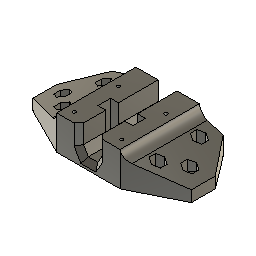
2Box Snare Int Bracket v1 (Autodesk Fusion 360 design; units mm, degrees)
Autodesk Fusion 360 part; units mm, degrees
sketch "Sketch1" plane through (0, 0, 0) normal (0, 0, 1) x (1, 0, 0)
  line L0 (0, 0) -> (40, 0)
  line L1 (40, 0) -> (40, 40)
  line L2 (40, 40) -> (0, 40)
  line L3 (0, 40) -> (0, 0)
  dimension "d1" = 40
  dimension "d2" = 40
  constraint horizontal L0
  constraint vertical L1
  constraint horizontal L2
  constraint vertical L3
  constraint coincident L0.start L3.end
  measures "d1" distance of L0.start L0.end
  measures "d2" distance of L0.start L2.end
extrude "Extrude1" add sketch "Sketch1" along normal blind 21.5
sketch "Sketch2" plane through (0, 0, 21.5) normal (0, 0, 1) x (-1, 0, 0)
  line L0 (0, -40) -> (0, 0)
  line L1 (0, 0) -> (-40, 0)
  line L2 (-40, 0) -> (-40, -40)
  line L3 (-40, -40) -> (0, -40)
  line L4 (-20, -55) -> (-20, 20) construction
  line L5 (-14.5, -40) -> (-25.5, -40)
  line L6 (-25.5, -40) -> (-25.5, 0)
  line L7 (-25.5, 0) -> (-14.5, 0)
  line L8 (-14.5, 0) -> (-14.5, -40)
  dimension "d5" = 20
  dimension "d6" = 11
  dimension "d7" = 5.5
  constraint perpendicular L3 L4
  constraint horizontal L5
  constraint vertical L6
  constraint horizontal L7
  constraint vertical L8
  constraint coincident L3 L5.start
  measures "d5" distance of L2 L4
  measures "d6" distance of L5.start L5.end
  measures "d7" distance of L4 L8
extrude "Extrude2" cut sketch "Sketch2" against normal blind 17 contours L1 L3 L5 L6 L7 L8
extrude "Extrude3" add 1 faces at (35.1667, 40, 8.6667) along direction (0, 1, 0) blind 10
sketch "Sketch3" plane through (0, 0, 0) normal (0, -1, 0) x (1, 0, 0)
  line L0 (25.5, 21.5) -> (25.5, 4.5)
  line L1 (25.5, 4.5) -> (14.5, 4.5)
  line L2 (14.5, 4.5) -> (14.5, 21.5)
  line L3 (14.5, 21.5) -> (0, 21.5)
  line L4 (0, 21.5) -> (0, 0)
  line L5 (0, 0) -> (40, 0)
  line L6 (40, 0) -> (40, 21.5)
  line L7 (40, 21.5) -> (25.5, 21.5)
  line L8 (13.9749, 9.6962) -> (16.9749, 4.5)
  line L9 (16.9749, 4.5) -> (22.9749, 4.5)
  line L10 (22.9749, 4.5) -> (25.9749, 9.6962)
  line L11 (14.5, 4.5) -> (30, 4.5) construction
  line L12 (25.9749, 9.6962) -> (25.9749, 21.5)
  line L13 (13.9749, 9.6962) -> (13.9749, 21.5)
  line L14 (13.9749, 21.5) -> (25.9749, 21.5)
  point P0 (19.9749, 9.6962)
  dimension "d13" = 12
  constraint coincident L1.end L2.start
  constraint perpendicular L2 L11
  constraint collinear L9 L11
  constraint coincident L7 L12.end
  constraint perpendicular L7 L12
  constraint coincident L3 L13.end
  constraint perpendicular L3 L13
  measures "d13" distance of L10.end L8.start
extrude "Extrude4" add 1 faces at (18.1667, 33.3333, 4.5) along direction (0, 0, 1) blind 17
extrude "Extrude5" cut sketch "Sketch3" against normal blind 61 contours L0 L7 L10 L12 L14 | L0 L1 L2 L8 L9 L10 L14 | L2 L3 L8 L13 L14
sketch "Sketch5" plane through (0, 0, 0) normal (0, 0, -1) x (1, 0, 0)
  line L0 (0, 0) -> (0, -50)
  line L1 (0, -50) -> (40, -50)
  line L2 (40, -50) -> (40, 0)
  line L3 (40, 0) -> (0, 0)
  circle A0 centre (20, -21) radius 4.5
  dimension "d19" = 9
  dimension "d20" = 21
  dimension "d21" = 20
  measures "d19" diameter of A0
  measures "d20" distance of L3 A0.centre
  measures "d21" distance of L2 A0.centre
extrude "Extrude6" cut sketch "Sketch5" against normal blind 51 contours A0
sketch "Sketch6" plane through (0, 0, 21.5) normal (0, 0, 1) x (-1, 0, 0)
  line L0 (-13.9749, 0) -> (-13.9749, -50)
  line L1 (-13.9749, -50) -> (0, -50)
  line L2 (0, -50) -> (0, 0)
  line L3 (0, 0) -> (-13.9749, 0)
  line L4 (-9, -25) -> (-31, -25)
  line L5 (-31, -25) -> (-31, -17)
  line L6 (-31, -17) -> (-9, -17)
  line L7 (-9, -17) -> (-9, -25)
  line L8 (-20, -32) -> (-20, 7) construction
  line L9 (4, -21) -> (-49, -21) construction
  dimension "d24" = 22
  dimension "d25" = 8
  dimension "d26" = 11
  dimension "d27" = 21
  dimension "d28" = 20
  dimension "d29" = 4
  constraint horizontal L4
  constraint vertical L5
  constraint horizontal L6
  constraint vertical L7
  constraint perpendicular L4 L8
  constraint perpendicular L5 L9
  measures "d24" distance of L4.start L4.end
  measures "d25" distance of L4.start L6.end
  measures "d26" distance of L7 L8
  measures "d27" distance of L3 L9
  measures "d28" distance of L2 L8
  measures "d29" distance of L4 L9
extrude "Extrude7" cut sketch "Sketch6" against normal blind 19 contours L0 L4 L6 L7 | L0 L4 L5 L6
sketch "Sketch7" plane through (0, 0, 0) normal (-1, 0, 0) x (0, -1, 0)
  line L0 (-50, 0) -> (0, 0)
  line L1 (0, 0) -> (0, 21.5)
  line L2 (0, 21.5) -> (-50, 21.5)
  line L3 (-50, 21.5) -> (-50, 0)
  line L4 (-50, 0) -> (0, 0)
  line L5 (0, 0) -> (0, 15)
  line L6 (0, 15) -> (-50, 15)
  line L7 (-50, 15) -> (-50, 0)
  constraint horizontal L4
  constraint vertical L5
  constraint horizontal L6
  constraint vertical L7
  constraint coincident L1 L5.end
  constraint coincident L0.start L3.end
extrude "Extrude8" add sketch "Sketch7" along normal blind 30 contours L0 L1 L3 L4 L5 L6 L7
sketch "Sketch8" plane through (40, 0, 0) normal (1, 0, 0) x (0, 1, 0)
  line L0 (0, 0) -> (50, 0)
  line L1 (50, 0) -> (50, 21.5)
  line L2 (50, 21.5) -> (0, 21.5)
  line L3 (0, 21.5) -> (0, 0)
  line L4 (0, 0) -> (50, 0)
  line L5 (50, 0) -> (50, 15)
  line L6 (50, 15) -> (0, 15)
  line L7 (0, 15) -> (0, 0)
  dimension "d34" = 50
  dimension "d35" = 15
  constraint horizontal L4
  constraint vertical L5
  constraint horizontal L6
  constraint vertical L7
  constraint coincident L0.start L3.end
  measures "d34" distance of L0.start L0.end
  measures "d35" distance of L0.start L6.end
extrude "Extrude9" add sketch "Sketch8" along normal blind 30 contours L0 L1 L3 L4 L5 L6 L7
sketch "Sketch9" plane through (0, 0, 15) normal (0, 0, 1) x (-1, 0, 0)
  line L0 (0, 0) -> (0, -50)
  line L1 (0, -50) -> (30, -50)
  line L2 (30, -50) -> (30, 0)
  line L3 (30, 0) -> (0, 0)
  line L4 (36, -15) -> (19, -15) construction
  line L5 (0, 0) -> (30, -15)
  line L6 (30, -30) -> (15, -50)
  line L7 (15, -50) -> (30, -50)
  line L8 (30, -50) -> (30, -30)
  line L9 (30, -15) -> (30, 0)
  line L10 (30, 0) -> (0, 0)
  line L11 (-70, -50) -> (-70, -30)
  line L12 (-70, -50) -> (-55, -50)
  line L13 (-55, -50) -> (-70, -30)
  line L14 (-70, 0) -> (-40, 0)
  line L15 (-70, 0) -> (-70, -15)
  line L16 (-70, -15) -> (-40, 0)
  dimension "d38" = 15
  dimension "d39" = 15
  dimension "d40" = 15
  dimension "d41" = 20
  dimension "d42" = 15
  dimension "d43" = 15
  constraint perpendicular L2 L4
  constraint coincident L0.start L3.end
  constraint coincident L4 L5.end
  constraint coincident L2 L5.end
  constraint coincident L1.end L2.start
  constraint coincident L2.end L3.start
  constraint perpendicular L10 L11
  constraint perpendicular L11 L12
  constraint perpendicular L11 L14
  constraint perpendicular L14 L15
  measures "d38" distance of L0.end L6.end
  measures "d39" distance of L3 L4
  measures "d40" distance of L5.end L6.start
  measures "d41" distance of L11.start L11.end
  measures "d42" distance of L11.start L12.end
  measures "d43" distance of L14.start L15.end
extrude "Extrude10" cut sketch "Sketch9" against normal blind 23 contours L2 L3 L5 L9 L10 | L1 L2 L6 L7 L8 | L11 L12 L13 | L14 L15 L16
sketch "Sketch10" plane through (0, 0, 21.5) normal (0, 0, 1) x (-1, 0, 0)
  line L0 (-9, -25) -> (-13.9749, -25)
  line L1 (-13.9749, -25) -> (-13.9749, -50)
  line L2 (-13.9749, -50) -> (0, -50)
  line L3 (0, -50) -> (0, 0)
  line L4 (0, 0) -> (-13.9749, 0)
  line L5 (-13.9749, 0) -> (-13.9749, -17)
  line L6 (-13.9749, -17) -> (-9, -17)
  line L7 (-9, -17) -> (-9, -25)
  point P0 (-5, -34)
  point P1 (-5, -6)
  point P2 (-35, -34)
  point P3 (-35, -6)
  dimension "d46" = 34
  dimension "d47" = 28
  dimension "d48" = 30
  dimension "d49" = 28
  dimension "d50" = 30
  dimension "d51" = 5
  measures "d46" distance of L4 P0
  measures "d47" distance of P0 P1
  measures "d48" distance of P0 P2
  measures "d49" vertical distance of P2 P3
  measures "d50" distance of P1 P3
  measures "d51" distance of L3 P0
hole "Hole1" at (5, 34, 21.5) at (35, 34, 21.5) at (35, 6, 21.5) at (5, 6, 21.5) direction (0, 0, -1) diameter 2 depth 18 tip angle 118
sketch "Sketch11" plane through (0, 0, 15) normal (0, 0, 1) x (-1, 0, 0)
  line L0 (15, -50) -> (30, -30)
  line L1 (30, -30) -> (30, -15)
  line L2 (30, -15) -> (0, 0)
  line L3 (0, 0) -> (0, -50)
  line L4 (0, -50) -> (15, -50)
  line L5 (-40, -50) -> (-55, -50)
  line L6 (-40, 0) -> (-40, -50)
  line L7 (-70, -30) -> (-70, -15)
  point P0 (10, -40)
  point P1 (20, -24)
  point P2 (10, -14)
  point P3 (-50, -40)
  point P4 (-60, -24)
  point P5 (-50, -14)
  dimension "d55" = 10
  dimension "d56" = 10
  dimension "d57" = 10
  dimension "d58" = 26
  dimension "d59" = 10
  dimension "d60" = 36
  dimension "d61" = 10
  dimension "d62" = 10
  dimension "d63" = 10
  dimension "d64" = 26
  dimension "d65" = 10
  dimension "d66" = 36
  measures "d55" distance of L4 P0
  measures "d56" distance of L3 P0
  measures "d57" distance of L1 P1
  measures "d58" distance of L4 P1
  measures "d59" distance of L3 P2
  measures "d60" distance of L4 P2
  measures "d61" distance of P3 L5
  measures "d62" distance of P3 L6
  measures "d63" distance of P4 L7
  measures "d64" distance of P4 L5
  measures "d65" distance of P5 L6
  measures "d66" distance of P5 L5
hole "Hole2" at (-10, 40, 15) at (-20, 24, 15) at (-10, 14, 15) at (50, 40, 15) at (60, 24, 15) at (50, 14, 15) direction (0, 0, -1) diameter 4 depth 18 tip angle 118
sketch "Sketch12" plane through (0, 0, 15) normal (0, 0, 1) x (-1, 0, 0)
  circle A0 centre (10, -14) radius 2
  circle A1 centre (10, -40) radius 2
  circle A2 centre (20, -24) radius 2
  line L0 (15, -50) -> (30, -30)
  line L1 (30, -30) -> (30, -15)
  line L2 (30, -15) -> (0, 0)
  line L3 (0, 0) -> (0, -50)
  line L4 (0, -50) -> (15, -50)
  line L5 (16.4, -26.0785) -> (20, -28.1569)
  line L6 (20, -28.1569) -> (23.6, -26.0785)
  line L7 (23.6, -26.0785) -> (23.6, -21.9215)
  line L8 (23.6, -21.9215) -> (20, -19.8431)
  line L9 (20, -19.8431) -> (16.4, -21.9215)
  line L10 (16.4, -21.9215) -> (16.4, -26.0785)
  line L11 (6.4, -42.0785) -> (10, -44.1569)
  line L12 (10, -44.1569) -> (13.6, -42.0785)
  line L13 (13.6, -42.0785) -> (13.6, -37.9215)
  line L14 (13.6, -37.9215) -> (10, -35.8431)
  line L15 (10, -35.8431) -> (6.4, -37.9215)
  line L16 (6.4, -37.9215) -> (6.4, -42.0785)
  line L17 (6.4, -16.0785) -> (10, -18.1569)
  line L18 (10, -18.1569) -> (13.6, -16.0785)
  line L19 (13.6, -16.0785) -> (13.6, -11.9215)
  line L20 (13.6, -11.9215) -> (10, -9.8431)
  line L21 (10, -9.8431) -> (6.4, -11.9215)
  line L22 (6.4, -11.9215) -> (6.4, -16.0785)
  line L23 (-53.6, -42.0785) -> (-50, -44.1569)
  line L24 (-50, -44.1569) -> (-46.4, -42.0785)
  line L25 (-46.4, -42.0785) -> (-46.4, -37.9215)
  line L26 (-46.4, -37.9215) -> (-50, -35.8431)
  line L27 (-50, -35.8431) -> (-53.6, -37.9215)
  line L28 (-53.6, -37.9215) -> (-53.6, -42.0785)
  line L29 (-63.6, -26.0785) -> (-60, -28.1569)
  line L30 (-60, -28.1569) -> (-56.4, -26.0785)
  line L31 (-56.4, -26.0785) -> (-56.4, -21.9215)
  line L32 (-56.4, -21.9215) -> (-60, -19.8431)
  line L33 (-60, -19.8431) -> (-63.6, -21.9215)
  line L34 (-63.6, -21.9215) -> (-63.6, -26.0785)
  line L35 (-53.6, -16.0785) -> (-50, -18.1569)
  line L36 (-50, -18.1569) -> (-46.4, -16.0785)
  line L37 (-46.4, -16.0785) -> (-46.4, -11.9215)
  line L38 (-46.4, -11.9215) -> (-50, -9.8431)
  line L39 (-50, -9.8431) -> (-53.6, -11.9215)
  line L40 (-53.6, -11.9215) -> (-53.6, -16.0785)
  point P0 (20, -24)
  point P1 (10, -40)
  point P2 (10, -14)
  point P3 (-50, -40)
  point P4 (-60, -24)
  point P5 (-50, -14)
  dimension "d70" = 3.6
  dimension "d71" = 3.6
  dimension "d72" = 3.6
  dimension "d73" = 3.6
  dimension "d74" = 3.6
  dimension "d75" = 3.6
  constraint coincident P0 A2.centre
  constraint coincident P1 A1.centre
  constraint coincident P2 A0.centre
  measures "d70" distance of P0 L10
  measures "d71" distance of P1 L16
  measures "d72" distance of P2 L22
  measures "d73" distance of P3 L28
  measures "d74" distance of P4 L34
  measures "d75" distance of P5 L40
extrude "Extrude11" cut sketch "Sketch12" against normal blind 10 contours L5 L6 L7 L8 L9 L10 | L11 L12 L13 L14 L15 L16 | L17 L18 L19 L20 L21 L22 | L23 L24 L25 L26 L27 L28 | L29 L30 L31 L32 L33 L34 | L35 L36 L37 L38 L39 L40
chamfer "Chamfer1" distance 8 distance2 25 2 edges at (-30, 22.5, 15) (70, 22.5, 15) measured on face at (-30, 25, 10) measured on face at (70, 20, 10)
fillet "Fillet1" radius 8 2 edges at (40, 25, 15) (0, 25, 15)
chamfer "Chamfer2" distance 3 angle 45 5 edges at (13.9749, 0, 15.5981) (15.4749, 0, 7.0981) (19.9749, 0, 4.5) (24.4749, 0, 7.0981) (25.9749, 0, 15.5981)
